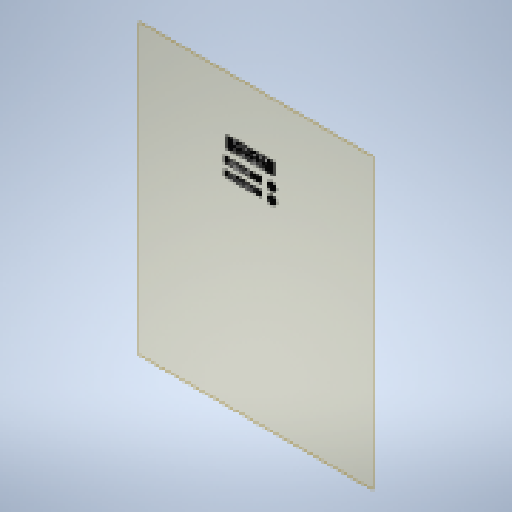
# Autodesk Inventor part: float-indicators
Saved by Autodesk Inventor 2023 (Build 270158030, 158C)
## iProperties
Created: 2024-04-02
Part Number: float-indicators
Material: Generic
Document SubType Name: Modeling
Designer: Imogen Heard
Density: 1 g/cm^3
Appearance: Default
Author: Imogen Heard
Autodesk Inventor part; units mm, degrees
ref_plane "YZ Plane" through (0, 0, 0) normal (1, 0, 0) x (0, 1, 0)
ref_plane "XZ Plane" through (0, 0, 0) normal (0, 1, 0) x (-1, 0, 0)
ref_plane "XY Plane" through (0, 0, 0) normal (0, 0, 1) x (1, 0, 0)
ref_plane "Work Plane1" through (0, 0, 0) normal (0, 0, 1) x (1, 0, 0)
sketch "Sketch1" plane through (0, 0, 0) normal (0, 0, 1) x (1, 0, 0)
  line L0 (-60.3338, 132.7229) -> (9.6662, 132.7229)
  line L1 (9.6662, 132.7229) -> (9.6662, 120.7229)
  line L2 (9.6662, 120.7229) -> (-60.3338, 120.7229)
  line L3 (-60.3338, 120.7229) -> (-60.3338, 132.7229)
  line L4 (-60.3338, 110.884) -> (9.6662, 110.884)
  line L5 (9.6662, 110.884) -> (9.6662, 98.884)
  line L6 (9.6662, 98.884) -> (-60.3338, 98.884)
  line L7 (-60.3338, 98.884) -> (-60.3338, 110.884)
  circle A0 centre (29.6662, 126.7229) radius 8
  circle A1 centre (29.6662, 126.7229) radius 10 construction
  circle A2 centre (29.6662, 104.884) radius 8
  circle A3 centre (29.6662, 104.884) radius 10 construction
  line L8 (-55.3338, 168.5239) -> (34.6662, 168.5239)
  line L9 (34.6662, 168.5239) -> (34.6662, 145.5239)
  line L10 (34.6662, 145.5239) -> (-55.3338, 145.5239)
  line L11 (-55.3338, 145.5239) -> (-55.3338, 168.5239)
  point P0 (0, 0)
  point P1 (9.6662, 104.884)
  point P2 (9.6662, 126.7229)
  dimension "d0" = 70
  dimension "d1" = 12
  dimension "d2" = 70
  dimension "d3" = 12
  dimension "d4" = 16
  dimension "d5" = 20
  dimension "d8" = 20
  dimension "d11" = 23
  dimension "d12" = 90
  dimension "d13" = 5
  constraints: 24 end point, 6 parallel, 4 centre point, 3 horizontal, 3 perpendicular, 2 equal radius, 2 horizontal alignment, 2 midpoint, 2 vertical alignment
  measures "d0" distance between parallel lines of L1 L3
  measures "d1" distance between parallel lines of L2 L0
  measures "d2" distance between parallel lines of L5 L7
  measures "d3" distance between parallel lines of L6 L4
  measures "d4" diameter of A0
  measures "d5" diameter of A1
  measures "d8" distance from line of L1 A0.centre
  measures "d11" distance between parallel lines of L10 L8
  measures "d12" distance between parallel lines of L9 L11
  measures "d13" distance between parallel lines of L11 L3
extrude "Extrusion1" add sketch "Sketch1" along normal blind 1
sketch "Sketch2" plane through (0, 0, 1) normal (0, 0, 1) x (1, 0, 0)
  line L0 (-42.3338, 167.5239) -> (21.8013, 167.5239) construction
  line L1 (21.8013, 167.5239) -> (21.8013, 146.5239) construction
  line L2 (21.8013, 146.5239) -> (-42.3338, 146.5239) construction
  line L3 (-42.3338, 146.5239) -> (-42.3338, 167.5239) construction
  line L4 (-55.3338, 145.5239) -> (34.6662, 145.5239) projected
  line L5 (34.6662, 168.5239) -> (-55.3338, 168.5239) projected
  line L6 (-55.3338, 168.5239) -> (-55.3338, 145.5239) projected
  point P0 (0, 0)
  dimension "d40" = 1
  dimension "d41" = 1
  dimension "d42" = 13
  constraints: 1 horizontal, 2 other
  measures "d40" distance between parallel lines of L4 L2
  measures "d41" distance between parallel lines of L5 L0
  measures "d42" distance between parallel lines of L6 L3
decal "Decal1"
sketch "Sketch3" plane through (0, 0, 1) normal (0, 0, 1) x (1, 0, 0)
  line L0 (-50.3338, 110.184) -> (-0.2783, 110.184) construction
  line L1 (-0.2783, 110.184) -> (-0.2783, 99.584) construction
  line L2 (-0.2783, 99.584) -> (-50.3338, 99.584) construction
  line L3 (-50.3338, 99.584) -> (-50.3338, 110.184) construction
  line L4 (9.6662, 132.7229) -> (-60.3338, 132.7229) projected
  line L5 (-60.3338, 120.7229) -> (9.6662, 120.7229) projected
  line L6 (-60.3338, 132.7229) -> (-60.3338, 120.7229) projected
  line L7 (-60.3338, 98.884) -> (9.6662, 98.884) projected
  line L8 (-60.3338, 110.884) -> (-60.3338, 98.884) projected
  line L9 (9.6662, 110.884) -> (-60.3338, 110.884) projected
  point P0 (0, 0)
  dimension "d58" = 0.7
  dimension "d59" = 10
  dimension "d60" = 0.7
  constraints: 1 horizontal, 2 other
  measures "d58" distance between parallel lines of L7 L2
  measures "d59" distance between parallel lines of L8 L3
  measures "d60" distance between parallel lines of L9 L0
decal "Decal2"
sketch "Sketch5" plane through (0, 0, 1) normal (0, 0, 1) x (1, 0, 0)
  line L0 (-50.3338, 132.0229) -> (-10.024, 132.0229) construction
  line L1 (-10.024, 132.0229) -> (-10.024, 121.4229) construction
  line L2 (-10.024, 121.4229) -> (-50.3338, 121.4229) construction
  line L3 (-50.3338, 121.4229) -> (-50.3338, 132.0229) construction
  line L4 (9.6662, 132.7229) -> (-60.3338, 132.7229) projected
  line L5 (-60.3338, 120.7229) -> (9.6662, 120.7229) projected
  line L6 (-60.3338, 132.7229) -> (-60.3338, 120.7229) projected
  point P0 (0, 0)
  dimension "d62" = 0.7
  dimension "d65" = 0.7
  dimension "d66" = 10
  constraints: 2 other
  measures "d62" distance between parallel lines of L4 L0
  measures "d65" distance between parallel lines of L5 L2
  measures "d66" distance between parallel lines of L6 L3
decal "Decal3"
body "Solid1"
